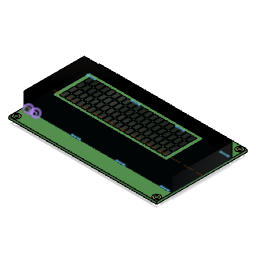
yeni_dash v3 (Autodesk Fusion 360 archive; units mm, degrees)
design "lcd"
Autodesk Fusion 360 part; units mm, degrees
note: some values were not read from the file. Chosen so that the rebuilt part matches the saved one: which bodies a step acts on; which face or edge a step refers to.
sketch "Sketch5" plane through (0, 0, 0) normal (0, 1, 0) x (1, 0, 0)
  line L0 (-49, 30) -> (49, 30)
  line L1 (49, 30) -> (49, -30)
  line L2 (49, -30) -> (-49, -30)
  line L3 (-49, -30) -> (-49, 30)
  dimension "d47" = 98
  dimension "d48" = 60
  constraint horizontal L0
  constraint vertical L1
  constraint horizontal L2
  constraint vertical L3
  measures "d47" distance of L0.start L0.end
  measures "d48" distance of L0.start L2.end
extrude "Extrude6" add sketch "Sketch5" along normal blind 1.6 makes body 1
sketch "Sketch6" plane through (0, 1.6, 0) normal (0, 1, 0) x (-1, 0, 0)
  line L0 (49, 30) -> (-49, 30)
  line L1 (-49, 30) -> (-49, -30)
  line L2 (-49, -30) -> (49, -30)
  line L3 (49, -30) -> (49, 30)
  circle A0 centre (46.5, -27.5) radius 2.25
  circle A1 centre (46.5, -27.5) radius 1.25
  line L4 (0, 0) -> (0, -40) construction
  line L5 (0, 0) -> (98, 0) construction
  circle A2 centre (-46.5, -27.5) radius 2.25
  circle A3 centre (-46.5, -27.5) radius 1.25
  circle A4 centre (46.5, 27.5) radius 2.25
  circle A5 centre (46.5, 27.5) radius 1.25
  circle A6 centre (-46.5, 27.5) radius 2.25
  circle A7 centre (-46.5, 27.5) radius 1.25
  circle A8 centre (39, -27) radius 0.4
  line L6 (49, 30) -> (49, -30)
  line L7 (49, -30) -> (-49, -30)
  arc A9 (40, -27) -> (38, -27) centre (39, -27) ccw
  line L8 (38, -27) -> (38, -30)
  line L9 (40, -27) -> (40, -30)
  line L10 (37.46, -27) -> (37.46, -30)
  circle A10 centre (36.46, -27) radius 0.4
  arc A11 (37.46, -27) -> (35.46, -27) centre (36.46, -27) ccw
  line L11 (35.46, -27) -> (35.46, -30)
  line L12 (34.92, -27) -> (34.92, -30)
  circle A12 centre (33.92, -27) radius 0.4
  arc A13 (34.92, -27) -> (32.92, -27) centre (33.92, -27) ccw
  line L13 (32.92, -27) -> (32.92, -30)
  line L14 (32.38, -27) -> (32.38, -30)
  circle A14 centre (31.38, -27) radius 0.4
  arc A15 (32.38, -27) -> (30.38, -27) centre (31.38, -27) ccw
  line L15 (30.38, -27) -> (30.38, -30)
  line L16 (29.84, -27) -> (29.84, -30)
  circle A16 centre (28.84, -27) radius 0.4
  arc A17 (29.84, -27) -> (27.84, -27) centre (28.84, -27) ccw
  line L17 (27.84, -27) -> (27.84, -30)
  line L18 (27.3, -27) -> (27.3, -30)
  circle A18 centre (26.3, -27) radius 0.4
  arc A19 (27.3, -27) -> (25.3, -27) centre (26.3, -27) ccw
  line L19 (25.3, -27) -> (25.3, -30)
  line L20 (24.76, -27) -> (24.76, -30)
  circle A20 centre (23.76, -27) radius 0.4
  arc A21 (24.76, -27) -> (22.76, -27) centre (23.76, -27) ccw
  line L21 (22.76, -27) -> (22.76, -30)
  line L22 (22.22, -27) -> (22.22, -30)
  circle A22 centre (21.22, -27) radius 0.4
  arc A23 (22.22, -27) -> (20.22, -27) centre (21.22, -27) ccw
  line L23 (20.22, -27) -> (20.22, -30)
  line L24 (19.68, -27) -> (19.68, -30)
  circle A24 centre (18.68, -27) radius 0.4
  arc A25 (19.68, -27) -> (17.68, -27) centre (18.68, -27) ccw
  line L25 (17.68, -27) -> (17.68, -30)
  line L26 (17.14, -27) -> (17.14, -30)
  circle A26 centre (16.14, -27) radius 0.4
  arc A27 (17.14, -27) -> (15.14, -27) centre (16.14, -27) ccw
  line L27 (15.14, -27) -> (15.14, -30)
  line L28 (14.6, -27) -> (14.6, -30)
  circle A28 centre (13.6, -27) radius 0.4
  arc A29 (14.6, -27) -> (12.6, -27) centre (13.6, -27) ccw
  line L29 (12.6, -27) -> (12.6, -30)
  line L30 (12.06, -27) -> (12.06, -30)
  circle A30 centre (11.06, -27) radius 0.4
  arc A31 (12.06, -27) -> (10.06, -27) centre (11.06, -27) ccw
  line L31 (10.06, -27) -> (10.06, -30)
  line L32 (9.52, -27) -> (9.52, -30)
  circle A32 centre (8.52, -27) radius 0.4
  arc A33 (9.52, -27) -> (7.52, -27) centre (8.52, -27) ccw
  line L33 (7.52, -27) -> (7.52, -30)
  line L34 (6.98, -27) -> (6.98, -30)
  circle A34 centre (5.98, -27) radius 0.4
  arc A35 (6.98, -27) -> (4.98, -27) centre (5.98, -27) ccw
  line L35 (4.98, -27) -> (4.98, -30)
  line L36 (4.44, -27) -> (4.44, -30)
  circle A36 centre (3.44, -27) radius 0.4
  arc A37 (4.44, -27) -> (2.44, -27) centre (3.44, -27) ccw
  line L37 (2.44, -27) -> (2.44, -30)
  line L38 (1.9, -27) -> (1.9, -30)
  circle A38 centre (0.9, -27) radius 0.4
  arc A39 (1.9, -27) -> (-0.1, -27) centre (0.9, -27) ccw
  line L39 (-0.1, -27) -> (-0.1, -30)
  line L40 (49, -20) -> (-49, -20)
  line L41 (-49, -20) -> (-49, 20)
  line L42 (-49, 20) -> (49, 20)
  line L43 (49, 20) -> (49, -20)
  dimension "d51" = 4.5
  dimension "d52" = 2.5
  dimension "d53" = 2.5
  dimension "d54" = 2.5
  dimension "d63" = 0.8
  dimension "d64" = 10
  dimension "d65" = 3
  dimension "d68" = -38.1
  dimension "d69" = 0
  dimension "d76" = 40
  constraint concentric A0 A1
  constraint coincident L4.start L5.start
  constraint perpendicular L2 L4
  constraint perpendicular L3 L5
  constraint symmetric A0 L4 A2
  constraint symmetric A1 L4 A3
  constraint symmetric A0 L5 A4
  constraint symmetric A1 L5 A5
  constraint symmetric L5 A2 A6
  constraint symmetric L5 A3 A7
  constraint coincident A8.centre A9.centre
  constraint coincident L7 L8.end
  constraint coincident L7 L9.end
  constraint horizontal L40
  constraint vertical L41
  constraint horizontal L42
  constraint vertical L43
  constraint coincident L1 L41.end
  constraint coincident L6 L40.start
  constraint midpoint L5 L43
  constraint midpoint L4 L40
  measures "d51" diameter of A0
  measures "d52" diameter of A1
  measures "d53" distance of L3 A0.centre
  measures "d54" distance of L2 A0.centre
  measures "d63" diameter of A8
  measures "d64" distance of A8.centre L6
  measures "d65" distance of A8.centre L7
  measures "d76" distance of L40.start L42.end
extrude "Extrude7" add sketch "Sketch6" along normal blind 0.1 contours A0 bodies 1
extrude "Extrude8" cut 1 faces at (-46.8443, 1.6, -27.3895) along direction (0, -1, 0) blind 2.2 on bodies 1 bodies 1
sketch "Sketch7" plane through (0, 1.7, 0) normal (0, 1, 0) x (-1, 0, 0)
  circle A0 centre (46.5, -27.5) radius 1.25
  circle A1 centre (46.5, -27.5) radius 2.25
extrude "Extrude9" add sketch "Sketch6" along normal blind 0.1 contours A2 | A4 | A6 bodies 1
extrude "Extrude10" cut sketch "Sketch6" against normal blind 3 contours A3 | A5 | A7 bodies 1
extrude "Extrude11" add sketch "Sketch6" along normal blind 0.1 contours L2 L7 A9 L8 L9 | L2 L7 L38 A39 L39 | L2 L7 L10 A11 L11 | L2 L7 L36 A37 L37 | L2 L7 L12 A13 L13 | L2 L7 L34 A35 L35 | L2 L7 L14 A15 L15 | L2 L7 L32 A33 L33 | L2 L7 L16 A17 L17 | L2 L7 L30 A31 L31 | L2 L7 L18 A19 L19 | L2 L7 L28 A29 L29 | L2 L7 L20 A21 L21 | L2 L7 L26 A27 L27 | L2 L7 L22 A23 L23 | L2 L7 L24 A25 L25 bodies 1
extrude "Extrude12" cut sketch "Sketch6" against normal blind 3 contours A8 | A10 | A12 | A14 | A16 | A18 | A20 | A22 | A24 | A26 | A28 | A30 | A32 | A34 | A36 | A38 bodies 1
extrude "Extrude13" add sketch "Sketch7" along normal blind 0.1 bodies 1
extrude "Extrude14" add sketch "Sketch6" along normal blind 9.4 contours L1 L3 L6 L40 L41 L42 L43 bodies 1
sketch "Sketch8" plane through (0, 11, 0) normal (0, 1, 0) x (-1, 0, 0)
  line L0 (49, 20) -> (-49, 20)
  line L1 (-49, 20) -> (-49, -20)
  line L2 (-49, -20) -> (49, -20)
  line L3 (49, -20) -> (49, 20)
  line L4 (0, 20) -> (0, -20) construction
  line L5 (0, 0) -> (98, 0)
  line L6 (-49, 0) -> (49, 0) construction
  line L7 (-38, -12.6) -> (38, -12.6)
  line L8 (38, -12.6) -> (38, 12.6)
  line L9 (38, 12.6) -> (-38, 12.6)
  line L10 (-38, 12.6) -> (-38, -12.6)
  dimension "d79" = 76
  dimension "d80" = 25.2
  dimension "d81" = 38
  dimension "d82" = 12.6
  constraint midpoint L0 L4.start
  constraint midpoint L2 L4.end
  constraint midpoint L1 L6.start
  constraint midpoint L5 L6.end
  constraint horizontal L7
  constraint vertical L8
  constraint horizontal L9
  constraint vertical L10
  measures "d79" distance of L7.start L7.end
  measures "d80" distance of L7.start L9.end
  measures "d81" distance of L4 L7.end
  measures "d82" distance of L6 L7.start
extrude "Extrude15" cut sketch "Sketch8" against normal blind 0.2 contours L7 L8 L9 L10 bodies 1
sketch "Sketch9" plane through (49, 0, 0) normal (1, 0, 0) x (0, 0, -1)
  line L0 (-30, 0) -> (30, 0)
  line L1 (30, 0) -> (30, 1.6)
  line L2 (30, 1.6) -> (20, 1.6)
  line L3 (20, 1.6) -> (20, 11)
  line L4 (20, 11) -> (-20, 11)
  line L5 (-20, 11) -> (-20, 1.6)
  line L6 (-20, 1.6) -> (-30, 1.6)
  line L7 (-30, 1.6) -> (-30, 0)
  line L8 (-20, 1.6) -> (20, 1.6)
  constraint coincident L5.end L6.start
  constraint coincident L2.end L3.start
split "Split1" by curves path "Sketch9" along L8 bodies 1 makes body 2 at (-18.69, 1.7, -29.133) makes body 3 at (-8.53, 1.7, -29.133) makes body 4 at (-21.23, 1.7, -29.133) makes body 5 at (-13.61, 1.7, -29.133) makes body 6 at (-28.85, 1.7, -29.133) makes body 7 at (-23.77, 1.7, -29.133) makes body 8 at (-31.39, 1.7, -29.133) makes body 9 at (-26.31, 1.7, -29.133) makes body 10 at (-33.93, 1.7, -29.133) makes body 11 at (-16.15, 1.7, -29.133) makes body 12 at (-36.47, 1.7, -29.133) makes body 13 at (-5.99, 1.7, -29.133) makes body 14 at (-39.01, 1.7, -29.133) makes body 15 at (44.5917, 1.7, 27.3882) makes body 16 at (-0.91, 1.7, -29.133) makes body 17 at (44.5917, 1.7, -27.6118) makes body 18 at (-3.45, 1.7, -29.133) makes body 19 at (-48.4083, 1.7, 27.3882) makes body 20 at (-48.4083, 1.8, -27.6118) makes body 21 at (-45.3333, 11, 0) makes body 22 at (-0.276, 0, 9.3536)
sketch "Sketch10" plane through (0, 10.8, 0) normal (0, 1, 0) x (-1, 0, 0)
  line L0 (-38, 12.6) -> (-38, -12.6)
  line L1 (-38, -12.6) -> (38, -12.6)
  line L2 (38, -12.6) -> (38, 12.6)
  line L3 (38, 12.6) -> (-38, 12.6)
  line L4 (0, 12.6) -> (0, -12.6) construction
  line L5 (38, 0) -> (-38, 0) construction
  line L6 (35.2, -10.4) -> (-35.2, -10.4) construction
  line L7 (-35.2, -10.4) -> (-35.2, 10.4) construction
  line L8 (-35.2, 10.4) -> (35.2, 10.4) construction
  line L9 (35.2, 10.4) -> (35.2, -10.4) construction
  line L10 (35.2, -10.4) -> (32.25, -10.4)
  line L11 (32.25, -10.4) -> (32.25, -5.65)
  line L12 (32.25, -5.65) -> (35.2, -5.65)
  line L13 (35.2, -5.65) -> (35.2, -10.4)
  line L14 (28.6974, -5.65) -> (31.6474, -5.65)
  line L15 (31.6474, -10.4) -> (28.6974, -10.4)
  line L16 (31.6474, -5.65) -> (31.6474, -10.4)
  line L17 (28.6974, -10.4) -> (28.6974, -5.65)
  line L18 (25.1447, -5.65) -> (28.0947, -5.65)
  line L19 (28.0947, -10.4) -> (25.1447, -10.4)
  line L20 (28.0947, -5.65) -> (28.0947, -10.4)
  line L21 (25.1447, -10.4) -> (25.1447, -5.65)
  line L22 (21.5921, -5.65) -> (24.5421, -5.65)
  line L23 (24.5421, -10.4) -> (21.5921, -10.4)
  line L24 (24.5421, -5.65) -> (24.5421, -10.4)
  line L25 (21.5921, -10.4) -> (21.5921, -5.65)
  line L26 (18.0395, -5.65) -> (20.9895, -5.65)
  line L27 (20.9895, -10.4) -> (18.0395, -10.4)
  line L28 (20.9895, -5.65) -> (20.9895, -10.4)
  line L29 (18.0395, -10.4) -> (18.0395, -5.65)
  line L30 (14.4868, -5.65) -> (17.4368, -5.65)
  line L31 (17.4368, -10.4) -> (14.4868, -10.4)
  line L32 (17.4368, -5.65) -> (17.4368, -10.4)
  line L33 (14.4868, -10.4) -> (14.4868, -5.65)
  line L34 (10.9342, -5.65) -> (13.8842, -5.65)
  line L35 (13.8842, -10.4) -> (10.9342, -10.4)
  line L36 (13.8842, -5.65) -> (13.8842, -10.4)
  line L37 (10.9342, -10.4) -> (10.9342, -5.65)
  line L38 (7.3816, -5.65) -> (10.3316, -5.65)
  line L39 (10.3316, -10.4) -> (7.3816, -10.4)
  line L40 (10.3316, -5.65) -> (10.3316, -10.4)
  line L41 (7.3816, -10.4) -> (7.3816, -5.65)
  line L42 (3.8289, -5.65) -> (6.7789, -5.65)
  line L43 (6.7789, -10.4) -> (3.8289, -10.4)
  line L44 (6.7789, -5.65) -> (6.7789, -10.4)
  line L45 (3.8289, -10.4) -> (3.8289, -5.65)
  line L46 (0.2763, -5.65) -> (3.2263, -5.65)
  line L47 (3.2263, -10.4) -> (0.2763, -10.4)
  line L48 (3.2263, -5.65) -> (3.2263, -10.4)
  line L49 (0.2763, -10.4) -> (0.2763, -5.65)
  line L50 (-3.2763, -5.65) -> (-0.3263, -5.65)
  line L51 (-0.3263, -10.4) -> (-3.2763, -10.4)
  line L52 (-0.3263, -5.65) -> (-0.3263, -10.4)
  line L53 (-3.2763, -10.4) -> (-3.2763, -5.65)
  line L54 (-6.8289, -5.65) -> (-3.8789, -5.65)
  line L55 (-3.8789, -10.4) -> (-6.8289, -10.4)
  line L56 (-3.8789, -5.65) -> (-3.8789, -10.4)
  line L57 (-6.8289, -10.4) -> (-6.8289, -5.65)
  line L58 (-10.3816, -5.65) -> (-7.4316, -5.65)
  line L59 (-7.4316, -10.4) -> (-10.3816, -10.4)
  line L60 (-7.4316, -5.65) -> (-7.4316, -10.4)
  line L61 (-10.3816, -10.4) -> (-10.3816, -5.65)
  line L62 (-13.9342, -5.65) -> (-10.9842, -5.65)
  line L63 (-10.9842, -10.4) -> (-13.9342, -10.4)
  line L64 (-10.9842, -5.65) -> (-10.9842, -10.4)
  line L65 (-13.9342, -10.4) -> (-13.9342, -5.65)
  line L66 (-17.4868, -5.65) -> (-14.5368, -5.65)
  line L67 (-14.5368, -10.4) -> (-17.4868, -10.4)
  line L68 (-14.5368, -5.65) -> (-14.5368, -10.4)
  line L69 (-17.4868, -10.4) -> (-17.4868, -5.65)
  line L70 (-21.0395, -5.65) -> (-18.0895, -5.65)
  line L71 (-18.0895, -10.4) -> (-21.0395, -10.4)
  line L72 (-18.0895, -5.65) -> (-18.0895, -10.4)
  line L73 (-21.0395, -10.4) -> (-21.0395, -5.65)
  line L74 (-24.5921, -5.65) -> (-21.6421, -5.65)
  line L75 (-21.6421, -10.4) -> (-24.5921, -10.4)
  line L76 (-21.6421, -5.65) -> (-21.6421, -10.4)
  line L77 (-24.5921, -10.4) -> (-24.5921, -5.65)
  line L78 (-28.1447, -5.65) -> (-25.1947, -5.65)
  line L79 (-25.1947, -10.4) -> (-28.1447, -10.4)
  line L80 (-25.1947, -5.65) -> (-25.1947, -10.4)
  line L81 (-28.1447, -10.4) -> (-28.1447, -5.65)
  line L82 (-31.6974, -5.65) -> (-28.7474, -5.65)
  line L83 (-28.7474, -10.4) -> (-31.6974, -10.4)
  line L84 (-28.7474, -5.65) -> (-28.7474, -10.4)
  line L85 (-31.6974, -10.4) -> (-31.6974, -5.65)
  line L86 (-35.25, -5.65) -> (-32.3, -5.65)
  line L87 (-32.3, -10.4) -> (-35.25, -10.4)
  line L88 (-32.3, -5.65) -> (-32.3, -10.4)
  line L89 (-35.25, -10.4) -> (-35.25, -5.65)
  line L90 (32.25, -0.3167) -> (35.2, -0.3167)
  line L91 (35.2, -5.0667) -> (32.25, -5.0667)
  line L92 (35.2, -0.3167) -> (35.2, -5.0667)
  line L93 (32.25, -5.0667) -> (32.25, -0.3167)
  line L94 (28.6974, -0.3167) -> (31.6474, -0.3167)
  line L95 (31.6474, -5.0667) -> (28.6974, -5.0667)
  line L96 (31.6474, -0.3167) -> (31.6474, -5.0667)
  line L97 (28.6974, -5.0667) -> (28.6974, -0.3167)
  line L98 (25.1447, -0.3167) -> (28.0947, -0.3167)
  line L99 (28.0947, -5.0667) -> (25.1447, -5.0667)
  line L100 (28.0947, -0.3167) -> (28.0947, -5.0667)
  line L101 (25.1447, -5.0667) -> (25.1447, -0.3167)
  line L102 (21.5921, -0.3167) -> (24.5421, -0.3167)
  line L103 (24.5421, -5.0667) -> (21.5921, -5.0667)
  line L104 (24.5421, -0.3167) -> (24.5421, -5.0667)
  line L105 (21.5921, -5.0667) -> (21.5921, -0.3167)
  line L106 (18.0395, -0.3167) -> (20.9895, -0.3167)
  line L107 (20.9895, -5.0667) -> (18.0395, -5.0667)
  line L108 (20.9895, -0.3167) -> (20.9895, -5.0667)
  line L109 (18.0395, -5.0667) -> (18.0395, -0.3167)
  line L110 (14.4868, -0.3167) -> (17.4368, -0.3167)
  line L111 (17.4368, -5.0667) -> (14.4868, -5.0667)
  line L112 (17.4368, -0.3167) -> (17.4368, -5.0667)
  line L113 (14.4868, -5.0667) -> (14.4868, -0.3167)
  line L114 (10.9342, -0.3167) -> (13.8842, -0.3167)
  line L115 (13.8842, -5.0667) -> (10.9342, -5.0667)
  line L116 (13.8842, -0.3167) -> (13.8842, -5.0667)
  line L117 (10.9342, -5.0667) -> (10.9342, -0.3167)
  line L118 (7.3816, -0.3167) -> (10.3316, -0.3167)
  line L119 (10.3316, -5.0667) -> (7.3816, -5.0667)
  line L120 (10.3316, -0.3167) -> (10.3316, -5.0667)
  line L121 (7.3816, -5.0667) -> (7.3816, -0.3167)
  line L122 (3.8289, -0.3167) -> (6.7789, -0.3167)
  line L123 (6.7789, -5.0667) -> (3.8289, -5.0667)
  line L124 (6.7789, -0.3167) -> (6.7789, -5.0667)
  line L125 (3.8289, -5.0667) -> (3.8289, -0.3167)
  line L126 (0.2763, -0.3167) -> (3.2263, -0.3167)
  line L127 (3.2263, -5.0667) -> (0.2763, -5.0667)
  line L128 (3.2263, -0.3167) -> (3.2263, -5.0667)
  line L129 (0.2763, -5.0667) -> (0.2763, -0.3167)
  line L130 (-3.2763, -0.3167) -> (-0.3263, -0.3167)
  line L131 (-0.3263, -5.0667) -> (-3.2763, -5.0667)
  line L132 (-0.3263, -0.3167) -> (-0.3263, -5.0667)
  line L133 (-3.2763, -5.0667) -> (-3.2763, -0.3167)
  line L134 (-6.8289, -0.3167) -> (-3.8789, -0.3167)
  line L135 (-3.8789, -5.0667) -> (-6.8289, -5.0667)
  line L136 (-3.8789, -0.3167) -> (-3.8789, -5.0667)
  line L137 (-6.8289, -5.0667) -> (-6.8289, -0.3167)
  line L138 (-10.3816, -0.3167) -> (-7.4316, -0.3167)
  line L139 (-7.4316, -5.0667) -> (-10.3816, -5.0667)
  line L140 (-7.4316, -0.3167) -> (-7.4316, -5.0667)
  line L141 (-10.3816, -5.0667) -> (-10.3816, -0.3167)
  line L142 (-13.9342, -0.3167) -> (-10.9842, -0.3167)
  line L143 (-10.9842, -5.0667) -> (-13.9342, -5.0667)
  line L144 (-10.9842, -0.3167) -> (-10.9842, -5.0667)
  line L145 (-13.9342, -5.0667) -> (-13.9342, -0.3167)
  line L146 (-17.4868, -0.3167) -> (-14.5368, -0.3167)
  line L147 (-14.5368, -5.0667) -> (-17.4868, -5.0667)
  line L148 (-14.5368, -0.3167) -> (-14.5368, -5.0667)
  line L149 (-17.4868, -5.0667) -> (-17.4868, -0.3167)
  line L150 (-21.0395, -0.3167) -> (-18.0895, -0.3167)
  line L151 (-18.0895, -5.0667) -> (-21.0395, -5.0667)
  line L152 (-18.0895, -0.3167) -> (-18.0895, -5.0667)
  line L153 (-21.0395, -5.0667) -> (-21.0395, -0.3167)
  line L154 (-24.5921, -0.3167) -> (-21.6421, -0.3167)
  line L155 (-21.6421, -5.0667) -> (-24.5921, -5.0667)
  line L156 (-21.6421, -0.3167) -> (-21.6421, -5.0667)
  line L157 (-24.5921, -5.0667) -> (-24.5921, -0.3167)
  line L158 (-28.1447, -0.3167) -> (-25.1947, -0.3167)
  line L159 (-25.1947, -5.0667) -> (-28.1447, -5.0667)
  line L160 (-25.1947, -0.3167) -> (-25.1947, -5.0667)
  line L161 (-28.1447, -5.0667) -> (-28.1447, -0.3167)
  line L162 (-31.6974, -0.3167) -> (-28.7474, -0.3167)
  line L163 (-28.7474, -5.0667) -> (-31.6974, -5.0667)
  line L164 (-28.7474, -0.3167) -> (-28.7474, -5.0667)
  line L165 (-31.6974, -5.0667) -> (-31.6974, -0.3167)
  line L166 (-35.25, -0.3167) -> (-32.3, -0.3167)
  line L167 (-32.3, -5.0667) -> (-35.25, -5.0667)
  line L168 (-32.3, -0.3167) -> (-32.3, -5.0667)
  line L169 (-35.25, -5.0667) -> (-35.25, -0.3167)
  line L170 (32.25, 5.0167) -> (35.2, 5.0167)
  line L171 (35.2, 0.2667) -> (32.25, 0.2667)
  line L172 (35.2, 5.0167) -> (35.2, 0.2667)
  line L173 (32.25, 0.2667) -> (32.25, 5.0167)
  line L174 (28.6974, 5.0167) -> (31.6474, 5.0167)
  line L175 (31.6474, 0.2667) -> (28.6974, 0.2667)
  line L176 (31.6474, 5.0167) -> (31.6474, 0.2667)
  line L177 (28.6974, 0.2667) -> (28.6974, 5.0167)
  line L178 (25.1447, 5.0167) -> (28.0947, 5.0167)
  line L179 (28.0947, 0.2667) -> (25.1447, 0.2667)
  line L180 (28.0947, 5.0167) -> (28.0947, 0.2667)
  line L181 (25.1447, 0.2667) -> (25.1447, 5.0167)
  line L182 (21.5921, 5.0167) -> (24.5421, 5.0167)
  line L183 (24.5421, 0.2667) -> (21.5921, 0.2667)
  line L184 (24.5421, 5.0167) -> (24.5421, 0.2667)
  line L185 (21.5921, 0.2667) -> (21.5921, 5.0167)
  line L186 (18.0395, 5.0167) -> (20.9895, 5.0167)
  line L187 (20.9895, 0.2667) -> (18.0395, 0.2667)
  line L188 (20.9895, 5.0167) -> (20.9895, 0.2667)
  line L189 (18.0395, 0.2667) -> (18.0395, 5.0167)
  line L190 (14.4868, 5.0167) -> (17.4368, 5.0167)
  line L191 (17.4368, 0.2667) -> (14.4868, 0.2667)
  line L192 (17.4368, 5.0167) -> (17.4368, 0.2667)
  line L193 (14.4868, 0.2667) -> (14.4868, 5.0167)
  line L194 (10.9342, 5.0167) -> (13.8842, 5.0167)
  line L195 (13.8842, 0.2667) -> (10.9342, 0.2667)
  line L196 (13.8842, 5.0167) -> (13.8842, 0.2667)
  line L197 (10.9342, 0.2667) -> (10.9342, 5.0167)
  line L198 (7.3816, 5.0167) -> (10.3316, 5.0167)
  line L199 (10.3316, 0.2667) -> (7.3816, 0.2667)
  line L200 (10.3316, 5.0167) -> (10.3316, 0.2667)
  line L201 (7.3816, 0.2667) -> (7.3816, 5.0167)
  line L202 (3.8289, 5.0167) -> (6.7789, 5.0167)
  line L203 (6.7789, 0.2667) -> (3.8289, 0.2667)
  line L204 (6.7789, 5.0167) -> (6.7789, 0.2667)
  line L205 (3.8289, 0.2667) -> (3.8289, 5.0167)
  line L206 (0.2763, 5.0167) -> (3.2263, 5.0167)
  line L207 (3.2263, 0.2667) -> (0.2763, 0.2667)
  line L208 (3.2263, 5.0167) -> (3.2263, 0.2667)
  line L209 (0.2763, 0.2667) -> (0.2763, 5.0167)
  line L210 (-3.2763, 5.0167) -> (-0.3263, 5.0167)
  line L211 (-0.3263, 0.2667) -> (-3.2763, 0.2667)
  line L212 (-0.3263, 5.0167) -> (-0.3263, 0.2667)
  line L213 (-3.2763, 0.2667) -> (-3.2763, 5.0167)
  line L214 (-6.8289, 5.0167) -> (-3.8789, 5.0167)
  line L215 (-3.8789, 0.2667) -> (-6.8289, 0.2667)
  line L216 (-3.8789, 5.0167) -> (-3.8789, 0.2667)
  line L217 (-6.8289, 0.2667) -> (-6.8289, 5.0167)
  line L218 (-10.3816, 5.0167) -> (-7.4316, 5.0167)
  line L219 (-7.4316, 0.2667) -> (-10.3816, 0.2667)
  line L220 (-7.4316, 5.0167) -> (-7.4316, 0.2667)
  line L221 (-10.3816, 0.2667) -> (-10.3816, 5.0167)
  line L222 (-13.9342, 5.0167) -> (-10.9842, 5.0167)
  line L223 (-10.9842, 0.2667) -> (-13.9342, 0.2667)
  line L224 (-10.9842, 5.0167) -> (-10.9842, 0.2667)
  line L225 (-13.9342, 0.2667) -> (-13.9342, 5.0167)
  line L226 (-17.4868, 5.0167) -> (-14.5368, 5.0167)
  line L227 (-14.5368, 0.2667) -> (-17.4868, 0.2667)
  line L228 (-14.5368, 5.0167) -> (-14.5368, 0.2667)
  line L229 (-17.4868, 0.2667) -> (-17.4868, 5.0167)
  line L230 (-21.0395, 5.0167) -> (-18.0895, 5.0167)
  line L231 (-18.0895, 0.2667) -> (-21.0395, 0.2667)
  line L232 (-18.0895, 5.0167) -> (-18.0895, 0.2667)
  line L233 (-21.0395, 0.2667) -> (-21.0395, 5.0167)
  line L234 (-24.5921, 5.0167) -> (-21.6421, 5.0167)
  line L235 (-21.6421, 0.2667) -> (-24.5921, 0.2667)
  line L236 (-21.6421, 5.0167) -> (-21.6421, 0.2667)
  line L237 (-24.5921, 0.2667) -> (-24.5921, 5.0167)
  line L238 (-28.1447, 5.0167) -> (-25.1947, 5.0167)
  line L239 (-25.1947, 0.2667) -> (-28.1447, 0.2667)
  line L240 (-25.1947, 5.0167) -> (-25.1947, 0.2667)
  line L241 (-28.1447, 0.2667) -> (-28.1447, 5.0167)
  line L242 (-31.6974, 5.0167) -> (-28.7474, 5.0167)
  line L243 (-28.7474, 0.2667) -> (-31.6974, 0.2667)
  line L244 (-28.7474, 5.0167) -> (-28.7474, 0.2667)
  line L245 (-31.6974, 0.2667) -> (-31.6974, 5.0167)
  line L246 (-35.25, 5.0167) -> (-32.3, 5.0167)
  line L247 (-32.3, 0.2667) -> (-35.25, 0.2667)
  line L248 (-32.3, 5.0167) -> (-32.3, 0.2667)
  line L249 (-35.25, 0.2667) -> (-35.25, 5.0167)
  line L250 (32.25, 10.35) -> (35.2, 10.35)
  line L251 (35.2, 5.6) -> (32.25, 5.6)
  line L252 (35.2, 10.35) -> (35.2, 5.6)
  line L253 (32.25, 5.6) -> (32.25, 10.35)
  line L254 (28.6974, 10.35) -> (31.6474, 10.35)
  line L255 (31.6474, 5.6) -> (28.6974, 5.6)
  line L256 (31.6474, 10.35) -> (31.6474, 5.6)
  line L257 (28.6974, 5.6) -> (28.6974, 10.35)
  line L258 (25.1447, 10.35) -> (28.0947, 10.35)
  line L259 (28.0947, 5.6) -> (25.1447, 5.6)
  line L260 (28.0947, 10.35) -> (28.0947, 5.6)
  line L261 (25.1447, 5.6) -> (25.1447, 10.35)
  line L262 (21.5921, 10.35) -> (24.5421, 10.35)
  line L263 (24.5421, 5.6) -> (21.5921, 5.6)
  line L264 (24.5421, 10.35) -> (24.5421, 5.6)
  line L265 (21.5921, 5.6) -> (21.5921, 10.35)
  line L266 (18.0395, 10.35) -> (20.9895, 10.35)
  line L267 (20.9895, 5.6) -> (18.0395, 5.6)
  line L268 (20.9895, 10.35) -> (20.9895, 5.6)
  line L269 (18.0395, 5.6) -> (18.0395, 10.35)
  line L270 (14.4868, 10.35) -> (17.4368, 10.35)
  line L271 (17.4368, 5.6) -> (14.4868, 5.6)
  line L272 (17.4368, 10.35) -> (17.4368, 5.6)
  line L273 (14.4868, 5.6) -> (14.4868, 10.35)
  line L274 (10.9342, 10.35) -> (13.8842, 10.35)
  line L275 (13.8842, 5.6) -> (10.9342, 5.6)
  line L276 (13.8842, 10.35) -> (13.8842, 5.6)
  line L277 (10.9342, 5.6) -> (10.9342, 10.35)
  line L278 (7.3816, 10.35) -> (10.3316, 10.35)
  line L279 (10.3316, 5.6) -> (7.3816, 5.6)
  line L280 (10.3316, 10.35) -> (10.3316, 5.6)
  line L281 (7.3816, 5.6) -> (7.3816, 10.35)
  line L282 (3.8289, 10.35) -> (6.7789, 10.35)
  line L283 (6.7789, 5.6) -> (3.8289, 5.6)
  line L284 (6.7789, 10.35) -> (6.7789, 5.6)
  line L285 (3.8289, 5.6) -> (3.8289, 10.35)
  line L286 (0.2763, 10.35) -> (3.2263, 10.35)
  line L287 (3.2263, 5.6) -> (0.2763, 5.6)
  line L288 (3.2263, 10.35) -> (3.2263, 5.6)
  line L289 (0.2763, 5.6) -> (0.2763, 10.35)
  line L290 (-3.2763, 10.35) -> (-0.3263, 10.35)
  line L291 (-0.3263, 5.6) -> (-3.2763, 5.6)
  line L292 (-0.3263, 10.35) -> (-0.3263, 5.6)
  line L293 (-3.2763, 5.6) -> (-3.2763, 10.35)
  line L294 (-6.8289, 10.35) -> (-3.8789, 10.35)
  line L295 (-3.8789, 5.6) -> (-6.8289, 5.6)
  line L296 (-3.8789, 10.35) -> (-3.8789, 5.6)
  line L297 (-6.8289, 5.6) -> (-6.8289, 10.35)
  line L298 (-10.3816, 10.35) -> (-7.4316, 10.35)
  line L299 (-7.4316, 5.6) -> (-10.3816, 5.6)
  line L300 (-7.4316, 10.35) -> (-7.4316, 5.6)
  line L301 (-10.3816, 5.6) -> (-10.3816, 10.35)
  line L302 (-13.9342, 10.35) -> (-10.9842, 10.35)
  line L303 (-10.9842, 5.6) -> (-13.9342, 5.6)
  line L304 (-10.9842, 10.35) -> (-10.9842, 5.6)
  line L305 (-13.9342, 5.6) -> (-13.9342, 10.35)
  line L306 (-17.4868, 10.35) -> (-14.5368, 10.35)
  line L307 (-14.5368, 5.6) -> (-17.4868, 5.6)
  line L308 (-14.5368, 10.35) -> (-14.5368, 5.6)
  line L309 (-17.4868, 5.6) -> (-17.4868, 10.35)
  line L310 (-21.0395, 10.35) -> (-18.0895, 10.35)
  line L311 (-18.0895, 5.6) -> (-21.0395, 5.6)
  line L312 (-18.0895, 10.35) -> (-18.0895, 5.6)
  line L313 (-21.0395, 5.6) -> (-21.0395, 10.35)
  line L314 (-24.5921, 10.35) -> (-21.6421, 10.35)
  line L315 (-21.6421, 5.6) -> (-24.5921, 5.6)
  line L316 (-21.6421, 10.35) -> (-21.6421, 5.6)
  line L317 (-24.5921, 5.6) -> (-24.5921, 10.35)
  line L318 (-28.1447, 10.35) -> (-25.1947, 10.35)
  line L319 (-25.1947, 5.6) -> (-28.1447, 5.6)
  line L320 (-25.1947, 10.35) -> (-25.1947, 5.6)
  line L321 (-28.1447, 5.6) -> (-28.1447, 10.35)
  line L322 (-31.6974, 10.35) -> (-28.7474, 10.35)
  line L323 (-28.7474, 5.6) -> (-31.6974, 5.6)
  line L324 (-28.7474, 10.35) -> (-28.7474, 5.6)
  line L325 (-31.6974, 5.6) -> (-31.6974, 10.35)
  line L326 (-35.25, 10.35) -> (-32.3, 10.35)
  line L327 (-32.3, 5.6) -> (-35.25, 5.6)
  line L328 (-32.3, 10.35) -> (-32.3, 5.6)
  line L329 (-35.25, 5.6) -> (-35.25, 10.35)
  dimension "d85" = 20.8
  dimension "d86" = 10.4
  dimension "d87" = 70.4
  dimension "d88" = 35.2
  dimension "d89" = 2.95
  dimension "d90" = 4.75
  dimension "d93" = -67.5
  dimension "d94" = 16
  constraint midpoint L3 L4.start
  constraint midpoint L1 L4.end
  constraint midpoint L2 L5.start
  constraint midpoint L0 L5.end
  constraint horizontal L6
  constraint vertical L7
  constraint horizontal L8
  constraint vertical L9
  constraint horizontal L10
  constraint vertical L11
  constraint horizontal L12
  constraint vertical L13
  measures "d85" distance of L6.start L8.end
  measures "d86" distance of L5 L6.start
  measures "d87" distance of L7.end L8.end
  measures "d88" distance of L4 L6.start
  measures "d89" distance of L6.start L10.end
  measures "d90" distance of L6.start L12.end
extrude "Extrude16" add sketch "Sketch10" along normal blind 0.05 separate body contours L10 L11 L12 L13 | L14 L15 L16 L17 | L18 L19 L20 L21 | L22 L23 L24 L25 | L26 L27 L28 L29 | L30 L31 L32 L33 | L34 L35 L36 L37 | L38 L39 L40 L41 | L42 L43 L44 L45 | L46 L47 L48 L49 | L50 L51 L52 L53 | L54 L55 L56 L57 | L58 L59 L60 L61 | L62 L63 L64 L65 | L66 L67 L68 L69 | L70 L71 L72 L73 | L74 L75 L76 L77 | L78 L79 L80 L81 | L82 L83 L84 L85 | L86 L87 L88 L89 | L90 L91 L92 L93 | L94 L95 L96 L97 | L98 L99 L100 L101 | L102 L103 L104 L105 | L106 L107 L108 L109 | L110 L111 L112 L113 | L114 L115 L116 L117 | L118 L119 L120 L121 | L122 L123 L124 L125 | L126 L127 L128 L129 | L130 L131 L132 L133 | L134 L135 L136 L137 | L138 L139 L140 L141 | L142 L143 L144 L145 | L146 L147 L148 L149 | L150 L151 L152 L153 | L154 L155 L156 L157 | L158 L159 L160 L161 | L162 L163 L164 L165 | L166 L167 L168 L169 | L170 L171 L172 L173 | L174 L175 L176 L177 | L178 L179 L180 L181 | L182 L183 L184 L185 | L186 L187 L188 L189 | L190 L191 L192 L193 | L194 L195 L196 L197 | L198 L199 L200 L201 | L202 L203 L204 L205 | L206 L207 L208 L209 | L210 L211 L212 L213 | L214 L215 L216 L217 | L218 L219 L220 L221 | L222 L223 L224 L225 | L226 L227 L228 L229 | L230 L231 L232 L233 | L234 L235 L236 L237 | L238 L239 L240 L241 | L242 L243 L244 L245 | L246 L247 L248 L249 | L250 L251 L252 L253 | L254 L255 L256 L257 | L258 L259 L260 L261 | L262 L263 L264 L265 | L266 L267 L268 L269 | L270 L271 L272 L273 | L274 L275 L276 L277 | L278 L279 L280 L281 | L282 L283 L284 L285 | L286 L287 L288 L289 | L290 L291 L292 L293 | L294 L295 L296 L297 | L298 L299 L300 L301 | L302 L303 L304 L305 | L306 L307 L308 L309 | L310 L311 L312 L313 | L314 L315 L316 L317 | L318 L319 L320 L321 | L322 L323 L324 L325 | L326 L327 L328 L329 makes body 23 at (27.1614, 10.8, 8.7667) makes body 24 at (12.9509, 10.8, 8.7667) makes body 25 at (30.714, 10.8, 3.4333) makes body 26 at (16.5035, 10.8, 3.4333) makes body 27 at (5.8456, 10.8, -1.9) makes body 28 at (20.0561, 10.8, -1.9) makes body 29 at (34.2667, 10.8, -3.4833) makes body 30 at (23.6088, 10.8, -7.2333) makes body 31 at (9.3982, 10.8, -7.2333) makes body 32 at (2.293, 10.8, 3.4333) makes body 33 at (-1.2596, 10.8, -1.9) makes body 34 at (-4.8123, 10.8, 3.4333) makes body 35 at (-9.3482, 10.8, -3.4833) makes body 36 at (-11.9175, 10.8, 3.4333) makes body 37 at (-15.4702, 10.8, -1.9) makes body 38 at (-22.5754, 10.8, -1.9) makes body 39 at (-19.0228, 10.8, 8.7667) makes body 40 at (-26.1281, 10.8, -1.9) makes body 41 at (-29.6807, 10.8, 3.4333) makes body 42 at (-33.2333, 10.8, -3.4833) makes body 43 at (-33.2333, 10.8, 1.85) makes body 44 at (-29.6807, 10.8, -1.9) makes body 45 at (-26.1281, 10.8, 3.4333) makes body 46 at (-22.5754, 10.8, 3.4333) makes body 47 at (-22.5754, 10.8, -7.2333) makes body 48 at (-15.4702, 10.8, 3.4333) makes body 49 at (-11.9175, 10.8, -1.9) makes body 50 at (-9.3482, 10.8, 1.85) makes body 51 at (-4.8123, 10.8, -1.9) makes body 52 at (-1.2596, 10.8, 3.4333) makes body 53 at (2.293, 10.8, -1.9) makes body 54 at (12.9509, 10.8, -7.2333) makes body 55 at (27.1614, 10.8, -7.2333) makes body 56 at (30.714, 10.8, -1.9) makes body 57 at (16.5035, 10.8, -1.9) makes body 58 at (5.8456, 10.8, 3.4333) makes body 59 at (20.0561, 10.8, 3.4333) makes body 60 at (34.2667, 10.8, 1.85) makes body 61 at (16.5035, 10.8, 8.7667) makes body 62 at (30.714, 10.8, 8.7667) makes body 63 at (23.6088, 10.8, 8.7667) makes body 64 at (9.3982, 10.8, 8.7667) makes body 65 at (27.1614, 10.8, 3.4333) makes body 66 at (12.9509, 10.8, 3.4333) makes body 67 at (9.3982, 10.8, -1.9) makes body 68 at (23.6088, 10.8, -1.9) makes body 69 at (34.2667, 10.8, -8.8167) makes body 70 at (20.0561, 10.8, -7.2333) makes body 71 at (5.8456, 10.8, -7.2333) makes body 72 at (2.293, 10.8, 8.7667) makes body 73 at (-1.2596, 10.8, -7.2333) makes body 74 at (-4.8123, 10.8, 8.7667) makes body 75 at (-8.3649, 10.8, -7.2333) makes body 76 at (-11.9175, 10.8, 8.7667) makes body 77 at (-15.4702, 10.8, -7.2333) makes body 78 at (-19.0228, 10.8, -1.9) makes body 79 at (-22.5754, 10.8, 8.7667) makes body 80 at (-26.1281, 10.8, -7.2333) makes body 81 at (-29.6807, 10.8, 8.7667) makes body 82 at (-33.2333, 10.8, -8.8167) makes body 83 at (-33.2333, 10.8, 7.1833) makes body 84 at (-29.6807, 10.8, -7.2333) makes body 85 at (-26.1281, 10.8, 8.7667) makes body 86 at (-19.0228, 10.8, 3.4333) makes body 87 at (-19.0228, 10.8, -7.2333) makes body 88 at (-15.4702, 10.8, 8.7667) makes body 89 at (-11.9175, 10.8, -7.2333) makes body 90 at (-9.3482, 10.8, 7.1833) makes body 91 at (-4.8123, 10.8, -7.2333) makes body 92 at (-1.2596, 10.8, 8.7667) makes body 93 at (2.293, 10.8, -7.2333) makes body 94 at (16.5035, 10.8, -7.2333) makes body 95 at (30.714, 10.8, -7.2333) makes body 96 at (27.1614, 10.8, -1.9) makes body 97 at (12.9509, 10.8, -1.9) makes body 98 at (9.3982, 10.8, 3.4333) makes body 99 at (23.6088, 10.8, 3.4333) makes body 100 at (5.8456, 10.8, 8.7667) makes body 101 at (20.0561, 10.8, 8.7667) makes body 102 at (34.2667, 10.8, 7.1833)
sketch "Sketch11" plane through (0, 0, 0) normal (0, -1, 0) x (1, 0, 0)
  circle A0 centre (-5.98, -27) radius 0.4
  circle A1 centre (-16.14, -27) radius 0.4
  circle A2 centre (-26.3, -27) radius 0.4
  circle A3 centre (-36.46, -27) radius 0.4
  circle A4 centre (-33.92, -27) radius 0.4
  circle A5 centre (-23.76, -27) radius 0.4
  circle A6 centre (-13.6, -27) radius 0.4
  circle A7 centre (-3.44, -27) radius 0.4
  circle A8 centre (-8.52, -27) radius 0.4
  circle A9 centre (-18.68, -27) radius 0.4
  circle A10 centre (-28.84, -27) radius 0.4
  circle A11 centre (-39, -27) radius 0.4
  circle A12 centre (-31.38, -27) radius 0.4
  circle A13 centre (-21.22, -27) radius 0.4
  circle A14 centre (-11.06, -27) radius 0.4
  circle A15 centre (-0.9, -27) radius 0.4
  circle A16 centre (-46.5, 27.5) radius 1.25
  circle A17 centre (46.5, -27.5) radius 1.25
  circle A18 centre (46.5, 27.5) radius 1.25
  circle A19 centre (-46.5, -27.5) radius 1.25
  line L0 (49, 30) -> (-49, 30)
  line L1 (-49, 30) -> (-49, -30)
  line L2 (-49, -30) -> (49, -30)
  line L3 (49, -30) -> (49, 30)
  line L4 (-49, 0) -> (49, 0) construction
  line L5 (-46.6, 19.1) -> (-41.8, 19.1)
  line L6 (-46.6, 20.3) -> (-41.8, 20.3)
  arc A20 (-46.6, 20.3) -> (-46.6, 19.1) centre (-46.6, 19.7) ccw
  arc A21 (-41.8, 19.1) -> (-41.8, 20.3) centre (-41.8, 19.7) ccw
  line L7 (47.2, 20.3) -> (47.2, 19.1) construction
  line L8 (-17.1333, 20.3) -> (-12.3333, 20.3)
  arc A22 (-17.1333, 20.3) -> (-17.1333, 19.1) centre (-17.1333, 19.7) ccw
  line L9 (-17.1333, 19.1) -> (-12.3333, 19.1)
  arc A23 (-12.3333, 19.1) -> (-12.3333, 20.3) centre (-12.3333, 19.7) ccw
  line L10 (12.3333, 20.3) -> (17.1333, 20.3)
  arc A24 (12.3333, 20.3) -> (12.3333, 19.1) centre (12.3333, 19.7) ccw
  line L11 (12.3333, 19.1) -> (17.1333, 19.1)
  arc A25 (17.1333, 19.1) -> (17.1333, 20.3) centre (17.1333, 19.7) ccw
  line L12 (41.8, 20.3) -> (46.6, 20.3)
  arc A26 (41.8, 20.3) -> (41.8, 19.1) centre (41.8, 19.7) ccw
  line L13 (41.8, 19.1) -> (46.6, 19.1)
  arc A27 (46.6, 19.1) -> (46.6, 20.3) centre (46.6, 19.7) ccw
  line L14 (-46.6, -20.3) -> (-41.8, -20.3)
  line L15 (-46.6, -19.1) -> (-41.8, -19.1)
  arc A28 (-46.6, -19.1) -> (-46.6, -20.3) centre (-46.6, -19.7) ccw
  arc A29 (-41.8, -20.3) -> (-41.8, -19.1) centre (-41.8, -19.7) ccw
  line L16 (-17.1333, -20.3) -> (-12.3333, -20.3)
  line L17 (-17.1333, -19.1) -> (-12.3333, -19.1)
  arc A30 (-17.1333, -19.1) -> (-17.1333, -20.3) centre (-17.1333, -19.7) ccw
  arc A31 (-12.3333, -20.3) -> (-12.3333, -19.1) centre (-12.3333, -19.7) ccw
  line L18 (12.3333, -20.3) -> (17.1333, -20.3)
  arc A32 (12.3333, -19.1) -> (12.3333, -20.3) centre (12.3333, -19.7) ccw
  line L19 (12.3333, -19.1) -> (17.1333, -19.1)
  arc A33 (17.1333, -20.3) -> (17.1333, -19.1) centre (17.1333, -19.7) ccw
  line L20 (41.8, -20.3) -> (46.6, -20.3)
  arc A34 (41.8, -19.1) -> (41.8, -20.3) centre (41.8, -19.7) ccw
  arc A35 (46.6, -20.3) -> (46.6, -19.1) centre (46.6, -19.7) ccw
  line L21 (41.8, -19.1) -> (46.6, -19.1)
  dimension "d109" = 88.4
  dimension "d110" = 0
  constraint midpoint L1 L4.start
  constraint midpoint L3 L4.end
  constraint symmetric L4 L5.start L15.start
  constraint symmetric L4 L5.end L15.end
  constraint symmetric L4 L6.start L14.start
  constraint symmetric L4 L6.end L14.end
  constraint symmetric L4 A20 A28
  constraint symmetric L4 A21 A29
  constraint symmetric L4 L8.start L16.start
  constraint symmetric L4 L8.end L16.end
  constraint symmetric L4 A22.end L17.start
  constraint symmetric L4 A22 A30
  constraint symmetric L4 L9.end L17.end
  constraint symmetric L4 A23 A31
  constraint symmetric L4 L10.start L18.start
  constraint symmetric L4 L10.end L18.end
  constraint symmetric L4 A24.end A32.start
  constraint symmetric L4 A24 A32
  constraint symmetric L4 L11.end L19.end
  constraint symmetric L4 A25 A33
  constraint symmetric L4 L12.start L20.start
  constraint symmetric L4 L12.end L20.end
  constraint symmetric L4 A26.end A34.start
  constraint symmetric L4 A26 A34
  constraint symmetric L4 L13.end A35.end
  constraint symmetric L4 A27 A35
extrude "Extrude17" cut sketch "Sketch11" against normal blind 1.6 contours L5 L6 A20 A21 | L8 A22 L9 A23 | L10 A24 L11 A25 | L12 A26 L13 A27 | L14 L15 A28 A29 | L16 L17 A30 A31 | L18 A32 L19 A33 | L20 A34 A35 L21 bodies 22
sketch "Sketch12" plane through (0, 1.6, 0) normal (0, -1, 0) x (1, 0, 0)
  line L0 (49, -20) -> (49, 20)
  line L1 (49, 20) -> (-49, 20)
  line L2 (-49, 20) -> (-49, -20)
  line L3 (-49, -20) -> (49, -20)
  line L4 (-46.6899, 20) -> (-41.6899, 20)
  line L5 (-41.6899, 20) -> (-41.6899, 19.5)
  line L6 (-41.6899, 19.5) -> (-46.6899, 19.5)
  line L7 (-46.6899, 19.5) -> (-46.6899, 20)
  arc A0 (-46.6, 20.3) -> (-46.6, 19.1) centre (-46.6, 19.7) ccw
  arc A1 (-41.8, 19.1) -> (-41.8, 20.3) centre (-41.8, 19.7) ccw
  line L8 (-47.2, 19.7) -> (-41.2, 19.7) construction
  line L9 (-46.6, 19.1) -> (-41.8, 19.1)
  line L10 (-46.6, 20.3) -> (-41.8, 20.3)
  line L11 (-44.2, 19.1) -> (-44.2, 20.3) construction
  line L12 (-17.2232, 20) -> (-12.2232, 20)
  line L13 (-17.2232, 19.5) -> (-17.2232, 20)
  line L14 (-12.2232, 19.5) -> (-17.2232, 19.5)
  line L15 (-12.2232, 20) -> (-12.2232, 19.5)
  line L16 (12.2435, 20) -> (17.2435, 20)
  line L17 (12.2435, 19.5) -> (12.2435, 20)
  line L18 (17.2435, 19.5) -> (12.2435, 19.5)
  line L19 (17.2435, 20) -> (17.2435, 19.5)
  line L20 (41.7101, 20) -> (46.7101, 20)
  line L21 (41.7101, 19.5) -> (41.7101, 20)
  line L22 (46.7101, 19.5) -> (41.7101, 19.5)
  line L23 (46.7101, 20) -> (46.7101, 19.5)
  line L24 (-49, 0) -> (49, 0) construction
  line L25 (41.7101, -20) -> (46.7101, -20)
  line L26 (46.7101, -19.5) -> (41.7101, -19.5)
  line L27 (41.7101, -19.5) -> (41.7101, -20)
  line L28 (46.7101, -20) -> (46.7101, -19.5)
  line L29 (17.2435, -20) -> (17.2435, -19.5)
  line L30 (12.2435, -20) -> (17.2435, -20)
  line L31 (17.2435, -19.5) -> (12.2435, -19.5)
  line L32 (12.2435, -19.5) -> (12.2435, -20)
  line L33 (-17.2232, -19.5) -> (-17.2232, -20)
  line L34 (-17.2232, -20) -> (-12.2232, -20)
  line L35 (-12.2232, -19.5) -> (-17.2232, -19.5)
  line L36 (-12.2232, -20) -> (-12.2232, -19.5)
  line L37 (-46.6899, -19.5) -> (-46.6899, -20)
  line L38 (-41.6899, -19.5) -> (-46.6899, -19.5)
  line L39 (-46.6899, -20) -> (-41.6899, -20)
  line L40 (-41.6899, -20) -> (-41.6899, -19.5)
  dimension "d113" = 5
  dimension "d114" = 0.5
  dimension "d117" = 88.4
  dimension "d118" = 0
  constraint horizontal L4
  constraint vertical L5
  constraint horizontal L6
  constraint vertical L7
  constraint coincident L1 L4.start
  constraint midpoint A0 L8.start
  constraint midpoint A1 L8.end
  constraint midpoint L9 L11.start
  constraint midpoint L10 L11.end
  constraint midpoint L2 L24.start
  constraint midpoint L0 L24.end
  constraint symmetric L4.start L24 L37.end
  constraint symmetric L4.end L24 L39.end
  constraint symmetric L5.end L24 L38.start
  constraint symmetric L6.end L24 L37.start
  constraint symmetric L12.start L24 L33.end
  constraint symmetric L12.end L24 L34.end
  constraint symmetric L13.start L24 L33.start
  constraint symmetric L14.start L24 L35.start
  constraint symmetric L16.start L24 L30.start
  constraint symmetric L16.end L24 L29.start
  constraint symmetric L17.start L24 L31.end
  constraint symmetric L18.start L24 L29.end
  constraint symmetric L20.start L24 L25.start
  constraint symmetric L20.end L24 L25.end
  constraint symmetric L21.start L24 L26.end
  constraint symmetric L22.start L24 L26.start
  measures "d113" distance of L4.start L4.end
  measures "d114" distance of L4.start L6.end
sketch "Sketch13" plane through (0, 0, 0) normal (0, -1, 0) x (1, 0, 0)
  line L0 (17.1333, -20.3) -> (12.3333, -20.3)
  arc A0 (12.3333, -19.1) -> (12.3333, -20.3) centre (12.3333, -19.7) ccw
  line L1 (12.3333, -19.1) -> (17.1333, -19.1)
  arc A1 (17.1333, -20.3) -> (17.1333, -19.1) centre (17.1333, -19.7) ccw
  line L2 (-12.3333, 19.1) -> (-17.1333, 19.1)
  arc A2 (-17.1333, 20.3) -> (-17.1333, 19.1) centre (-17.1333, 19.7) ccw
  line L3 (-17.1333, 20.3) -> (-12.3333, 20.3)
  arc A3 (-12.3333, 19.1) -> (-12.3333, 20.3) centre (-12.3333, 19.7) ccw
  line L4 (17.1333, 19.1) -> (12.3333, 19.1)
  arc A4 (12.3333, 20.3) -> (12.3333, 19.1) centre (12.3333, 19.7) ccw
  line L5 (12.3333, 20.3) -> (17.1333, 20.3)
  arc A5 (17.1333, 19.1) -> (17.1333, 20.3) centre (17.1333, 19.7) ccw
  line L6 (-12.3333, -20.3) -> (-17.1333, -20.3)
  arc A6 (-17.1333, -19.1) -> (-17.1333, -20.3) centre (-17.1333, -19.7) ccw
  line L7 (-17.1333, -19.1) -> (-12.3333, -19.1)
  arc A7 (-12.3333, -20.3) -> (-12.3333, -19.1) centre (-12.3333, -19.7) ccw
  arc A8 (46.6, -20.3) -> (46.6, -19.1) centre (46.6, -19.7) ccw
  line L8 (46.6, -20.3) -> (41.8, -20.3)
  arc A9 (41.8, -19.1) -> (41.8, -20.3) centre (41.8, -19.7) ccw
  line L9 (41.8, -19.1) -> (46.6, -19.1)
  line L10 (-41.8, 19.1) -> (-46.6, 19.1)
  arc A10 (-46.6, 20.3) -> (-46.6, 19.1) centre (-46.6, 19.7) ccw
  line L11 (-46.6, 20.3) -> (-41.8, 20.3)
  arc A11 (-41.8, 19.1) -> (-41.8, 20.3) centre (-41.8, 19.7) ccw
  line L12 (46.6, 19.1) -> (41.8, 19.1)
  arc A12 (41.8, 20.3) -> (41.8, 19.1) centre (41.8, 19.7) ccw
  line L13 (41.8, 20.3) -> (46.6, 20.3)
  arc A13 (46.6, 19.1) -> (46.6, 20.3) centre (46.6, 19.7) ccw
  line L14 (-41.8, -20.3) -> (-46.6, -20.3)
  arc A14 (-46.6, -19.1) -> (-46.6, -20.3) centre (-46.6, -19.7) ccw
  line L15 (-46.6, -19.1) -> (-41.8, -19.1)
  arc A15 (-41.8, -20.3) -> (-41.8, -19.1) centre (-41.8, -19.7) ccw
  circle A16 centre (-5.98, -27) radius 0.4
  circle A17 centre (-16.14, -27) radius 0.4
  circle A18 centre (-26.3, -27) radius 0.4
  circle A19 centre (-36.46, -27) radius 0.4
  circle A20 centre (-33.92, -27) radius 0.4
  circle A21 centre (-23.76, -27) radius 0.4
  circle A22 centre (-13.6, -27) radius 0.4
  circle A23 centre (-3.44, -27) radius 0.4
  circle A24 centre (-8.52, -27) radius 0.4
  circle A25 centre (-18.68, -27) radius 0.4
  circle A26 centre (-28.84, -27) radius 0.4
  circle A27 centre (-39, -27) radius 0.4
  circle A28 centre (-31.38, -27) radius 0.4
  circle A29 centre (-21.22, -27) radius 0.4
  circle A30 centre (-11.06, -27) radius 0.4
  circle A31 centre (-0.9, -27) radius 0.4
  circle A32 centre (-46.5, 27.5) radius 1.25
  circle A33 centre (46.5, -27.5) radius 1.25
  circle A34 centre (46.5, 27.5) radius 1.25
  circle A35 centre (-46.5, -27.5) radius 1.25
  line L16 (49, 30) -> (-49, 30)
  line L17 (-49, 30) -> (-49, -30)
  line L18 (-49, -30) -> (49, -30)
  line L19 (49, -30) -> (49, 30)
extrude "Extrude18" add sketch "Sketch12" along normal blind 4 contours L1 L4 L5 L6 L7 bodies 21
extrude "Extrude19" add sketch "Sketch12" along normal blind 4 contours L1 L12 L13 L14 L15 bodies 21
extrude "Extrude20" add sketch "Sketch12" along normal blind 4 contours L1 L16 L17 L18 L19 bodies 21
extrude "Extrude21" add sketch "Sketch12" along normal blind 4 contours L1 L20 L21 L22 L23 bodies 21
extrude "Extrude22" add sketch "Sketch12" along normal blind 4 contours L3 L37 L38 L39 L40 bodies 21
extrude "Extrude23" add sketch "Sketch12" along normal blind 4 contours L3 L33 L34 L35 L36 bodies 21
extrude "Extrude24" add sketch "Sketch12" along normal blind 4 contours L3 L29 L30 L31 L32 bodies 21
extrude "Extrude25" add sketch "Sketch12" along normal blind 4 contours L3 L25 L26 L27 L28 bodies 21
equation "d53 = ( ( 98 - 93 ) / 2 ) * 1 mm"
equation "d54 = ( ( 60 - 55 ) / 2 ) * 1 mm"
equation "d81 = ( 76 / 2 ) * 1 mm"
equation "d82 = ( 25.2 / 2 ) * 1 mm"
equation "d86 = ( 20.8 / 2 ) * 1 mm"
equation "d88 = ( 70.4 / 2 ) * 1 mm"
